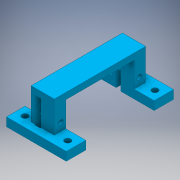
# Autodesk Inventor part: MotorHolder_forM
Saved by Autodesk Inventor 2018.2 (Build 222227000, 227)
## iProperties
Created: 2017-09-28
Part Number: MotorHolder_forM
Material: ナイロン 6/6
Document SubType Name: Modeling
Designer: sktom
Density: 1.13 g/cm^3
Appearance: スカイ ブルー 標準
Author: sktom
Autodesk Inventor part; units mm, degrees
ref_plane "YZ Plane" through (0, 0, 0) normal (1, 0, 0) x (0, 1, 0)
ref_plane "XZ Plane" through (0, 0, 0) normal (0, 1, 0) x (-1, 0, 0)
ref_plane "XY Plane" through (0, 0, 0) normal (0, 0, 1) x (1, 0, 0)
sketch "スケッチ1" plane through (0, 0, 0) normal (0, 0, 1) x (1, 0, 0)
  line L0 (4.7874, 3.074) -> (-2.4126, 3.074) construction
  line L1 (-2.4126, 3.074) -> (-2.4126, -2.5626) construction
  line L2 (4.6566, -2.5626) -> (-2.4126, -2.5626) construction
  line L3 (4.6566, -14.1826) -> (4.6566, -2.5626) construction
  line L4 (32.7567, -14.1826) -> (4.6566, -14.1826) construction
  arc A0 (33.6403, -15.0662) -> (32.7567, -14.1826) centre (32.7567, -15.0662) ccw construction
  line L5 (33.6403, -15.0662) -> (33.6403, -5.3461) construction
  arc A1 (32.7567, -6.2297) -> (33.6403, -5.3461) centre (32.7567, -5.3461) ccw construction
  line L6 (32.7567, -6.2297) -> (28.4268, -6.2297) construction
  line L7 (28.4268, 12.9897) -> (28.4268, -6.2297) construction
  line L8 (28.4268, 12.9897) -> (33.7287, 12.9897) construction
  line L9 (33.7287, 34.374) -> (33.7287, 12.9897) construction
  line L10 (-2.4126, 34.374) -> (33.7287, 34.374) construction
  line L11 (-2.4126, 34.374) -> (-2.4126, 27.674) construction
  line L12 (-2.4126, 27.674) -> (4.7874, 27.674) construction
  line L13 (4.7874, 27.674) -> (4.7874, 31.674) construction
  line L14 (4.7874, 31.674) -> (7.0874, 31.674) construction
  line L15 (7.0874, 31.674) -> (7.0874, 27.674) construction
  line L16 (7.0874, 27.674) -> (22.5874, 27.674) construction
  line L17 (22.5874, 27.674) -> (22.5874, 3.074) construction
  line L18 (22.5874, 3.074) -> (7.0874, 3.074) construction
  line L19 (7.0874, 3.074) -> (7.0874, -0.926) construction
  line L20 (7.0874, -0.926) -> (4.7874, -0.926) construction
  line L21 (4.7874, -0.926) -> (4.7874, 3.074) construction
  line L22 (4.9614, 30.124) -> (6.5614, 30.124) construction
  line L23 (4.9614, 28.124) -> (6.5614, 28.124) construction
  line L24 (6.5614, 27.174) -> (20.8114, 27.174) construction
  line L25 (6.5614, 29.374) -> (6.5614, 31.374) construction
  line L26 (6.5614, 26.174) -> (6.5614, 29.374) construction
  line L27 (18.4524, 3.574) -> (6.5614, 3.574) construction
  line L28 (6.5614, 1.374) -> (6.5614, 4.574) construction
  line L29 (6.5614, -0.626) -> (6.5614, 1.374) construction
  line L30 (4.9614, 2.624) -> (6.5614, 2.624) construction
  line L31 (4.9614, 0.624) -> (6.5614, 0.624) construction
  line L32 (6.5614, 31.374) -> (18.5614, 31.374)
  line L33 (18.5614, 31.374) -> (18.5614, -0.626)
  line L34 (18.5614, -0.626) -> (6.5614, -0.626)
  line L35 (6.5614, -0.626) -> (6.5614, 31.374)
  circle A2 centre (0.5874, 30.674) radius 0.8
  circle A3 centre (15.5614, 0.074) radius 0.8
  circle A4 centre (0.5874, 0.074) radius 0.8
  circle A5 centre (15.5614, 30.674) radius 0.8
  point P0 (0, 0)
extrude "押し出し1" add sketch "スケッチ1" along normal blind 14 contours L32 A5 L33 L34 A3 L35 | L32 A5 | A3 L34 picked at (15.5843, 30.875) picked at (15.5358, 0.3268)
sketch "スケッチ2" plane through (6.5614, -0.626, 0) normal (-1, 0, 0) x (0, 0, 1)
  line L0 (1, 27.8) -> (10.6, 27.8) construction
  arc A0 (11.6, 26.8) -> (10.6, 27.8) centre (10.6, 26.8) ccw construction
  line L1 (11.6, 26.8) -> (11.6, 30) construction
  arc A1 (11.6, 30) -> (9.6, 32) centre (9.6, 30) ccw construction
  line L2 (2, 32) -> (9.6, 32) construction
  arc A2 (2, 32) -> (0, 30) centre (2, 30) ccw construction
  line L3 (0, 26.8) -> (0, 30) construction
  arc A3 (1, 27.8) -> (0, 26.8) centre (1, 26.8) ccw construction
  circle A4 centre (5.8, 29.75) radius 1 construction
  arc A5 (10.6, 4.2) -> (11.6, 5.2) centre (10.6, 5.2) ccw construction
  line L4 (10.6, 4.2) -> (1, 4.2) construction
  arc A6 (0, 5.2) -> (1, 4.2) centre (1, 5.2) ccw construction
  line L5 (0, 2) -> (0, 5.2) construction
  arc A7 (0, 2) -> (2, 0) centre (2, 2) ccw construction
  line L6 (9.6, 0) -> (2, 0) construction
  arc A8 (9.6, 0) -> (11.6, 2) centre (9.6, 2) ccw construction
  line L7 (11.6, 2) -> (11.6, 5.2) construction
  circle A9 centre (5.8, 2.25) radius 1 construction
  circle A10 centre (5.8, 29.75) radius 0.85
  circle A11 centre (5.8, 2.25) radius 0.85
  point P0 (0, 0.626)
  dimension "d3" = 1.7
  constraints: 2 centre point, 2 coincident, 1 equal radius
  measures "d3" diameter of A10
extrude "押し出し2" cut sketch "スケッチ2" against normal up to next
sketch "スケッチ3" plane through (6.5614, -0.626, 0) normal (-1, 0, 0) x (0, 0, 1)
  line L0 (9.6, 27.8) -> (2, 27.8) construction
  line L1 (11.6, 9.918) -> (11.6, 25.8) construction
  spline S0 degree 5 poles (31.6664, 3.8342) (33.0444, 2.9064) (34.3681, 1.8973) (35.6334, 0.8093) (37.4433, -0.9431) (39.0884, -2.8469) (39.625, -3.5071) (40.1413, -4.1828) (40.6369, -4.8737) knots 0.500883 0.500883 0.500883 0.500883 0.500883 0.500883 16.687593 16.687593 16.687593 24.970224 24.970224 24.970224 24.970224 24.970224 24.970224 construction
  line L2 (1, 27.8) -> (10.6, 27.8) construction
  arc A0 (11.6, 26.8) -> (10.6, 27.8) centre (10.6, 26.8) ccw construction
  line L3 (11.6, 26.8) -> (11.6, 30) construction
  arc A1 (11.6, 30) -> (9.6, 32) centre (9.6, 30) ccw construction
  line L4 (2, 32) -> (9.6, 32) construction
  arc A2 (2, 32) -> (0, 30) centre (2, 30) ccw construction
  line L5 (0, 26.8) -> (0, 30) construction
  arc A3 (1, 27.8) -> (0, 26.8) centre (1, 26.8) ccw construction
  circle A4 centre (5.8, 29.75) radius 1 construction
  arc A5 (10.6, 4.2) -> (11.6, 5.2) centre (10.6, 5.2) ccw construction
  line L6 (10.6, 4.2) -> (1, 4.2) construction
  arc A6 (0, 5.2) -> (1, 4.2) centre (1, 5.2) ccw construction
  line L7 (0, 2) -> (0, 5.2) construction
  arc A7 (0, 2) -> (2, 0) centre (2, 2) ccw construction
  line L8 (9.6, 0) -> (2, 0) construction
  arc A8 (9.6, 0) -> (11.6, 2) centre (9.6, 2) ccw construction
  line L9 (11.6, 2) -> (11.6, 5.2) construction
  circle A9 centre (5.8, 2.25) radius 1 construction
  line L10 (11.8, 28) -> (-0.2, 28)
  line L11 (-0.2, 28) -> (-0.2, 4)
  line L12 (-0.2, 4) -> (11.8, 4)
  line L13 (11.8, 4) -> (11.8, 28)
  line L14 (0, 0) -> (0, 32) projected
  point P0 (0, 0.626)
  dimension "d6" = 0.2
  dimension "d7" = 0.2
  dimension "d8" = 0.2
  dimension "d9" = 0.2
  constraints: 8 end point, 2 parallel, 1 horizontal, 1 perpendicular
  measures "d6" distance between parallel lines of L13 L1
  measures "d7" distance from line of L6.start L12
  measures "d8" distance between parallel lines of L2 L10
  measures "d9" distance between parallel lines of L14 L11
extrude "押し出し3" cut sketch "スケッチ3" against normal up to next
sketch "スケッチ4" plane through (6.5614, 31.374, 0) normal (0, 1, 0) x (1, 0, 0)
  line L0 (12, -14) -> (0, -14) projected
  line L1 (12, -14) -> (5, -14)
  line L2 (5, -14) -> (5, -3)
  line L3 (5, -3) -> (12, -3)
  line L4 (12, -3) -> (12, -14)
  line L5 (0, 0) -> (12, 0) projected
  point P0 (-6.5614, 0)
  dimension "d12" = 7
  dimension "d13" = 3
  constraints: 8 end point, 2 parallel, 1 horizontal, 1 perpendicular
  measures "d12" distance of L2.end L3.end
  measures "d13" distance between parallel lines of L5 L3
extrude "押し出し4" cut sketch "スケッチ4" against normal up to next
sketch "スケッチ5" plane through (6.5614, -0.626, 0) normal (0, -1, 0) x (1, 0, 0)
  line L0 (12, 0) -> (12, 3) projected
  line L1 (12, 3) -> (0, 3)
  line L2 (0, 3) -> (0, 0)
  line L3 (0, 0) -> (12, 0)
  line L4 (12, 0) -> (12, 3)
  point P0 (-6.5614, 0)
  constraints: 8 end point, 2 parallel, 1 coincident, 1 horizontal, 1 perpendicular
extrude "押し出し5" add sketch "スケッチ5" along normal blind 2.8
sketch "スケッチ6" plane through (6.5614, 31.374, 0) normal (0, 1, 0) x (1, 0, 0)
  line L0 (12, -3) -> (0, -3) projected
  line L1 (0, 0) -> (0, -14) projected
  line L2 (12, -3) -> (0, -3)
  line L3 (0, -3) -> (0, 0)
  line L4 (0, 0) -> (12, 0)
  line L5 (12, 0) -> (12, -3)
  point P0 (-6.5614, 0)
  constraints: 8 end point, 2 parallel, 1 horizontal, 1 perpendicular
extrude "押し出し6" add sketch "スケッチ6" along normal blind 2.8
sketch "スケッチ7" plane through (0, 0, 0) normal (0, 0, -1) x (-1, 0, 0)
  line L0 (-4.7874, 3.074) -> (2.4126, 3.074) construction
  line L1 (2.4126, 3.074) -> (2.4126, -2.5626) construction
  line L2 (-4.6566, -2.5626) -> (2.4126, -2.5626) construction
  line L3 (-4.6566, -14.1826) -> (-4.6566, -2.5626) construction
  line L4 (-32.7567, -14.1826) -> (-4.6566, -14.1826) construction
  arc A0 (-32.7567, -14.1826) -> (-33.6403, -15.0662) centre (-32.7567, -15.0662) ccw construction
  line L5 (-33.6403, -15.0662) -> (-33.6403, -5.3461) construction
  arc A1 (-33.6403, -5.3461) -> (-32.7567, -6.2297) centre (-32.7567, -5.3461) ccw construction
  line L6 (-32.7567, -6.2297) -> (-28.4268, -6.2297) construction
  line L7 (-28.4268, 12.9897) -> (-28.4268, -6.2297) construction
  line L8 (-28.4268, 12.9897) -> (-33.7287, 12.9897) construction
  line L9 (-33.7287, 34.374) -> (-33.7287, 12.9897) construction
  line L10 (2.4126, 34.374) -> (-33.7287, 34.374) construction
  line L11 (2.4126, 34.374) -> (2.4126, 27.674) construction
  line L12 (2.4126, 27.674) -> (-4.7874, 27.674) construction
  line L13 (-4.7874, 27.674) -> (-4.7874, 31.674) construction
  line L14 (-4.7874, 31.674) -> (-7.0874, 31.674) construction
  line L15 (-7.0874, 31.674) -> (-7.0874, 27.674) construction
  line L16 (-7.0874, 27.674) -> (-22.5874, 27.674) construction
  line L17 (-22.5874, 27.674) -> (-22.5874, 3.074) construction
  line L18 (-22.5874, 3.074) -> (-7.0874, 3.074) construction
  line L19 (-7.0874, 3.074) -> (-7.0874, -0.926) construction
  line L20 (-7.0874, -0.926) -> (-4.7874, -0.926) construction
  line L21 (-4.7874, -0.926) -> (-4.7874, 3.074) construction
  line L22 (-4.9614, 31.374) -> (-4.9614, 29.374) construction
  line L23 (-6.9374, 3.074) -> (-6.9374, -0.926) construction
  line L24 (-22.5874, 3.074) -> (-7.0874, 3.074) construction
  line L25 (-22.4374, 27.674) -> (-22.4374, 3.074) construction
  line L26 (-7.0874, 27.674) -> (-22.5874, 27.674) construction
  line L27 (-6.9374, 31.674) -> (-6.9374, 27.674) construction
  line L28 (-4.7874, 31.674) -> (-7.0874, 31.674) construction
  line L29 (-4.6374, 27.674) -> (-4.6374, 31.674) construction
  line L30 (2.4126, 27.674) -> (-4.7874, 27.674) construction
  line L31 (2.5626, 3.074) -> (2.5626, 27.674) construction
  line L32 (-4.7874, 3.074) -> (2.4126, 3.074) construction
  line L33 (-4.6374, -0.926) -> (-4.6374, 3.074) construction
  line L34 (-7.0874, -0.926) -> (-4.7874, -0.926) construction
  line L35 (-4.9614, 1.374) -> (-4.9614, -0.626) construction
  line L36 (-6.5614, 27.374) -> (-6.5614, 34.174) projected
  line L37 (-6.5614, 34.174) -> (2.4126, 34.174)
  line L38 (2.4126, 34.174) -> (2.4126, 27.674)
  line L39 (2.4126, 27.674) -> (-4.9614, 27.674)
  line L40 (-4.9614, 27.674) -> (-4.9614, 31.674)
  line L41 (-4.9614, 31.674) -> (-6.5614, 31.674)
  line L42 (-6.5614, 31.674) -> (-6.5614, 34.174)
  line L43 (-6.5614, -0.626) -> (-6.5614, -3.426) projected
  line L44 (-6.5614, -3.426) -> (2.4126, -3.426)
  line L45 (2.4126, -3.426) -> (2.4126, 3.074)
  line L46 (2.4126, 3.074) -> (-4.9614, 3.074)
  line L47 (-4.9614, 3.074) -> (-4.9614, -0.926)
  line L48 (-4.9614, -0.926) -> (-6.5614, -0.926)
  line L49 (-6.5614, -0.926) -> (-6.5614, -3.426)
  circle A2 centre (-0.5874, 30.674) radius 0.8 projected
  circle A3 centre (-15.5614, 0.074) radius 0.8 projected
  circle A4 centre (-0.5874, 0.074) radius 0.8 projected
  circle A5 centre (-15.5614, 30.674) radius 0.8 projected
  point P0 (0, 0)
  constraints: 24 end point, 8 point on line, 5 collinear, 4 perpendicular, 1 horizontal, 1 parallel
extrude "押し出し7" add sketch "スケッチ7" against normal up to surface (3 mm away) contours L36 L37 L38 L39 L40 L41 | L48 L47 L46 L45 L44 L43 | A2 | A4
sketch "スケッチ8" plane through (6.5614, 31.374, 3) normal (0, 0, 1) x (1, 0, 0)
  line L0 (-8.974, -28.3) -> (-1.6, -28.3) projected
  line L1 (-1.6, -32) -> (-3.1, -32)
  line L2 (-3.1, -32) -> (-3.1, -28.3)
  line L3 (-3.1, -28.3) -> (-1.6, -28.3)
  line L4 (-1.6, -28.3) -> (-1.6, -32)
  line L5 (-1.6, -32.3) -> (-1.6, -28.3) projected
  line L6 (0, -32) -> (5, -32) projected
  line L7 (-1.6, -3.7) -> (-8.974, -3.7) projected
  line L8 (-1.6, 0) -> (-3.1, 0)
  line L9 (-3.1, 0) -> (-3.1, -3.7)
  line L10 (-3.1, -3.7) -> (-1.6, -3.7)
  line L11 (-1.6, -3.7) -> (-1.6, 0)
  line L12 (5, 0) -> (0, 0) projected
  line L13 (-1.6, -3.7) -> (-1.6, 0.3) projected
  point P0 (-6.5614, -31.374)
  dimension "d22" = 1.5
  constraints: 16 end point, 4 collinear, 4 parallel, 3 point on line, 2 horizontal, 2 perpendicular
  measures "d22" distance of L1.start L1.end
extrude "押し出し8" add sketch "スケッチ8" along normal up to surface (11 mm away)
sketch "スケッチ9" plane through (0, 0, 14) normal (0, 0, 1) x (1, 0, 0)
  line L0 (11.5614, -0.626) -> (11.5614, 31.374) construction
  line L1 (11.5614, 31.374) -> (6.5614, 31.374) construction
  line L2 (6.5614, 31.374) -> (6.5614, -0.626) construction
  line L3 (6.5614, -0.626) -> (11.5614, -0.626) construction
  line L4 (4.9614, 31.374) -> (4.9614, 27.674) construction
  line L5 (3.4614, 31.374) -> (4.9614, 31.374) construction
  line L6 (3.4614, 27.674) -> (3.4614, 31.374) construction
  line L7 (4.9614, 27.674) -> (3.4614, 27.674) construction
  line L8 (4.9614, -0.626) -> (3.4614, -0.626) construction
  line L9 (4.9614, 3.074) -> (4.9614, -0.626) construction
  line L10 (3.4614, 3.074) -> (4.9614, 3.074) construction
  line L11 (3.4614, -0.626) -> (3.4614, 3.074) construction
  line L12 (6.5614, 31.374) -> (4.9614, 31.374)
  line L13 (4.9614, 31.374) -> (4.9614, 27.674)
  line L14 (4.9614, 27.674) -> (3.4614, 27.674) projected
  line L15 (4.9614, 27.674) -> (3.4614, 27.674)
  line L16 (3.4614, -0.626) -> (3.4614, 3.074) projected
  line L17 (3.4614, 27.674) -> (3.4614, 3.074)
  line L18 (3.4614, 3.074) -> (4.9614, 3.074)
  line L19 (4.9614, -0.626) -> (3.4614, -0.626) projected
  line L20 (4.9614, 3.074) -> (4.9614, -0.626)
  line L21 (4.9614, -0.626) -> (6.5614, -0.626)
  line L22 (6.5614, -0.626) -> (6.5614, 31.374)
  point P0 (0, 0)
  constraints: 16 end point, 4 perpendicular, 3 collinear, 1 horizontal
extrude "押し出し9" add sketch "スケッチ9" against normal up to surface (2.2 mm away) contours L22 L21 L20 L18 L17 L14 L13 L12
sketch "スケッチ10" plane through (3.4614, 27.674, 3) normal (-1, 0, 0) x (0, 0, 1)
  circle A0 centre (2.8, 1.45) radius 0.85 construction
  circle A1 centre (2.8, -26.05) radius 1 construction
  circle A2 centre (2.8, 1.45) radius 1
  circle A3 centre (2.8, -26.05) radius 1
  point P0 (-3, -27.674)
  dimension "d27" = 2
  constraints: 2 centre point, 2 coincident, 1 equal radius
  measures "d27" diameter of A2
extrude "押し出し10" cut sketch "スケッチ10" against normal up to next
sketch "スケッチ11" plane through (6.5614, 31.374, 3) normal (0, 0, 1) x (1, 0, 0)
  circle A0 centre (9, -0.7) radius 1.05
  circle A1 centre (-5.974, -0.7) radius 1.05
  line L0 (-8.974, 2.8) -> (-8.974, -3.7) projected
  line L1 (-8.974, -3.7) -> (-3.1, -3.7) projected
  line L2 (12, -4) -> (12, 2.8) projected
  circle A2 centre (9, -31.3) radius 1.05
  circle A3 centre (-5.974, -31.3) radius 1.05
  line L3 (-3.1, -28.3) -> (-8.974, -28.3) projected
  point P0 (-6.5614, -31.374)
  dimension "d30" = 3
  dimension "d31" = 3
  dimension "d32" = 2.1
  dimension "d33" = 3
  dimension "d34" = 3
  constraints: 4 centre point, 3 equal radius, 2 horizontal alignment, 2 vertical alignment
  measures "d30" distance from line of A1.centre L0
  measures "d31" distance from line of A1.centre L1
  measures "d32" diameter of A1
  measures "d33" distance from line of L2 A0.centre
  measures "d34" distance from line of L3 A3.centre
extrude "押し出し11" cut sketch "スケッチ11" against normal up to next
sketch "スケッチ12" plane through (0, 0, 0) normal (0, 0, -1) x (-1, 0, 0)
  line L0 (-6.5614, 31.674) -> (-4.9614, 31.674) projected
  line L1 (-18.5614, 27.374) -> (-6.5614, 27.374) projected
  line L2 (-6.5614, 31.674) -> (-6.8614, 31.674)
  line L3 (-6.8614, 31.674) -> (-6.8614, 27.374)
  line L4 (-6.8614, 27.374) -> (-6.5614, 27.374)
  line L5 (-6.5614, 27.374) -> (-6.5614, 31.674)
  line L6 (-4.9614, -0.926) -> (-6.5614, -0.926) projected
  line L7 (-6.5614, -0.926) -> (-6.8614, -0.926)
  line L8 (-6.8614, -0.926) -> (-6.8614, 3.374)
  line L9 (-6.8614, 3.374) -> (-6.5614, 3.374)
  line L10 (-6.5614, 3.374) -> (-6.5614, -0.926)
  line L11 (-6.5614, 3.374) -> (-18.5614, 3.374) projected
  point P0 (0, 0)
  dimension "d37" = 0.3
  constraints: 16 end point, 4 parallel, 2 horizontal, 2 perpendicular, 2 point on line, 1 collinear
  measures "d37" distance between parallel lines of L5 L3
extrude "押し出し12" cut sketch "スケッチ12" against normal up to surface (11.8 mm away)
